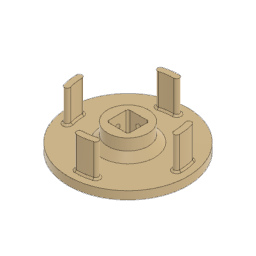
spool adapter v11 (Autodesk Fusion 360 design; units mm, degrees)
Autodesk Fusion 360 part; units mm, degrees
note: some values were not read from the file. Set by a fixed rule: which sketch regions a step uses.
sketch "Sketch1" plane through (0, 0, 0) normal (0, 0, 1) x (1, 0, 0)
  circle A0 centre (0, 0) radius 36.75
  dimension "d1" = 73.5
  constraint coincident A0.centre origin
  measures "d1" diameter of A0
extrude "Extrude1" add sketch "Sketch1" along normal blind 5
sketch "Sketch3" plane through (0, 0, 5) normal (0, 0, 1) x (-1, 0, 0)
  circle A0 centre (0, 0) radius 36.75
  circle A1 centre (0, 0) radius 30 construction
  line L0 (0, 0) -> (-30, 0) construction
  arc A2 (-31.75, 0) -> (-30.3627, -9.2828) centre (0, 0) ccw
  arc A3 (-28.25, 0) -> (-31.75, 0) centre (-30, 0) ccw
  arc A4 (-28.25, 0) -> (-27.0156, -8.2595) centre (0, 0) ccw
  arc A5 (-30.3627, -9.2828) -> (-27.0156, -8.2595) centre (-28.6891, -8.7712) ccw
  arc A6 (-30, 0) -> (-28.6891, -8.7712) centre (0, 0) ccw construction
  dimension "d8" = 60
  dimension "d24" = 3.5
  dimension "d27" = 17
  constraint coincident A0.centre A1.centre
  constraint coincident A1 L0.end
  constraint horizontal L0
  constraint tangent A2 A3
  constraint tangent A3 A4
  constraint tangent A4 A5
  constraint tangent A2 A5
  constraint coincident L0.end A3.centre
  measures "d8" diameter of A1
  measures "d24" distance of A2 A4
  measures "d27" angle of A5.centre L0.end A0.centre
extrude "Extrude3" add sketch "Sketch3" along normal blind 20 contours A2 A3 A4 A5
chamfer "Chamfer2" distance 1 angle 45 4 edges at (27.9397, 4.1756, 5) (28.1775, 10.4447, 5) (31.4013, 4.6929, 5) (30, -1.75, 5)
pattern_circular "C-Pattern1" count 4 over 360 about axis through (0, 0, 1.75) along (0, 0, 1) of "Extrude3", "Chamfer2"
sketch "Sketch4" plane through (0, 0, 5) normal (0, 0, 1) x (-1, 0, 0)
  circle A0 centre (0, 0) radius 12.5
  arc A1 (27.25, 0) -> (26.0593, 7.9671) centre (0, 0) ccw
  arc A2 (31.319, 9.5752) -> (26.0593, 7.9671) centre (28.6891, 8.7712) ccw
  arc A3 (27.25, 0) -> (32.75, 0) centre (30, 0) ccw
  arc A4 (-27.25, 0) -> (-26.0593, -7.9671) centre (0, 0) ccw
  arc A5 (-31.319, -9.5752) -> (-26.0593, -7.9671) centre (-28.6891, -8.7712) ccw
  arc A6 (-27.25, 0) -> (-32.75, 0) centre (-30, 0) ccw
  arc A7 (0, -27.25) -> (7.9671, -26.0593) centre (0, 0) ccw
  arc A8 (9.5752, -31.319) -> (7.9671, -26.0593) centre (8.7712, -28.6891) ccw
  arc A9 (0, -27.25) -> (0, -32.75) centre (0, -30) ccw
  arc A10 (0, 27.25) -> (-7.9671, 26.0593) centre (0, 0) ccw
  arc A11 (-9.5752, 31.319) -> (-7.9671, 26.0593) centre (-8.7712, 28.6891) ccw
  arc A12 (0, 27.25) -> (0, 32.75) centre (0, 30) ccw
  arc A13 (32.75, 0) -> (31.319, 9.5752) centre (0, 0) ccw
  arc A14 (-32.75, 0) -> (-31.319, -9.5752) centre (0, 0) ccw
  circle A15 centre (0, 0) radius 36.75
  arc A16 (0, -32.75) -> (9.5752, -31.319) centre (0, 0) ccw
  arc A17 (0, 32.75) -> (-9.5752, 31.319) centre (0, 0) ccw
  dimension "d14" = 25
  constraint coincident A0.centre A1.centre
  measures "d14" diameter of A0
extrude "Extrude4" add sketch "Sketch4" along normal blind 11 contours A0
sketch "Sketch5" plane through (0, 0, 0) normal (0, 0, -1) x (1, 0, 0)
  circle A0 centre (0, 0) radius 36.75
  line L0 (6.6, -6.6) -> (-6.6, -6.6)
  line L1 (-6.6, -6.6) -> (-6.6, 6.6)
  line L2 (-6.6, 6.6) -> (6.6, 6.6)
  line L3 (6.6, 6.6) -> (6.6, -6.6)
  line L4 (6.6, -6.6) -> (-6.6, 6.6) construction
  line L5 (-6.6, -6.6) -> (6.6, 6.6) construction
  dimension "d17" = 13.2
  dimension "d18" = 13.2
  constraint perpendicular L0 L1
  constraint parallel L0 L2
  constraint parallel L1 L3
  constraint horizontal L0
  constraint coincident L4 A0.centre
  constraint coincident L5 A0.centre
  constraint coincident A0.centre origin
  measures "d17" distance of L0.end L1.end
  measures "d18" distance of L1.end L2.end
extrude "Extrude5" cut sketch "Sketch5" against normal up to surface (16 mm away) contours L0 L1 L2 L3
sketch "Sketch9" plane through (6.5, 0, 0) normal (-1, 0, 0) x (0, -1, 0)
  line L0 (6.5, 19) -> (-6.5, 19)
  line L1 (-6.5, 19) -> (-6.5, 0)
  line L2 (-6.5, 0) -> (6.5, 0)
  line L3 (6.5, 0) -> (6.5, 19)
  line L4 (0, 0) -> (0, 11.85)
  circle A0 centre (0, 9.6) radius 2.25
  dimension "d53" = 9.6
  dimension "d54" = 4.5
  constraint coincident L4.start origin
  constraint perpendicular L2 L4
  constraint coincident L4 A0.centre
  constraint coincident L4.end A0
  measures "d53" distance of L4.start A0.centre
  measures "d54" diameter of A0
revolve "Revolve2" [suppressed]
pattern_circular "C-Pattern3" [suppressed]
sketch "Sketch8" plane through (0, 0, 0) normal (0, 0, -1) x (1, 0, 0)
  line L0 (6.6, 6.6) -> (6.6, -6.6)
  line L1 (6.6, -6.6) -> (-6.6, -6.6)
  line L2 (-6.6, -6.6) -> (-6.6, 6.6)
  line L3 (-6.6, 6.6) -> (6.6, 6.6)
  circle A0 centre (0, 0) radius 36.75
  circle A1 centre (0, 0) radius 7.75
  dimension "d49" = 15.5
  constraint coincident A0.centre A1.centre
  measures "d49" diameter of A1
extrude "Extrude8" cut sketch "Sketch8" against normal blind 10 draft -30 contours L0 A1 | L0 L1 L2 L3 A1 | L3 A1 | L1 A1 | L2 A1
fillet "Fillet2" radius 1.3 4 edges at (-6.6, 6.6, 8) (6.6, -6.6, 8) (-6.6, -6.6, 8) (6.6, 6.6, 8)
chamfer "Chamfer1" distance 4 angle 45 1 edges at (11.6541, -4.5202, 5)
ref_plane "WorkPlane1" through (5.6, 0, 8) normal (-1, 0, 0) x (0, -1, 0)
sketch "Sketch10" plane through (5.6, 0, 9.5) normal (-1, 0, 0) x (0, 1, 0)
  line L0 (5.3, -6.5) -> (5.3, 9.5)
  line L1 (5.3, 9.5) -> (4.0623, 9.5)
  spline S0 degree 2 poles (4.0623, 9.5) (0, 5.8118) (-4.0623, 9.5) knots 0 0 0 0.904876 0.904876 0.904876 weights 1 1.174242 1
  line L2 (-4.0623, 9.5) -> (-5.3, 9.5)
  line L3 (-5.3, 9.5) -> (-5.3, -6.5)
  line L4 (-5.3, -6.5) -> (5.3, -6.5)
  spline S1 degree 2 poles (4.0623, 9.5) (0, 5.8118) (-4.0623, 9.5) knots 0 0 0 0.904876 0.904876 0.904876 weights 1 1.174242 1
  line L5 (-4.0623, 9.5) -> (4.0623, 9.5)
  line L6 (0, 9.5) -> (0, -6.5)
  circle A0 centre (0, 0) radius 2
  dimension "d60" = 4
  dimension "d61" = 9.5
  constraint midpoint L5 L6.start
  constraint midpoint L4 L6.end
  constraint coincident L6 A0.centre
  measures "d60" diameter of A0
  measures "d61" distance of L5 A0.centre
revolve "Revolve3" cut sketch "Sketch10" angle 360 about axis through (5.6, 0, 0) along (0, 0, 1) contours L6 A0 picked at (0.5315, 0.497)
pattern_circular "C-Pattern4" count 4 over 360 about axis through (0, 0, 1.75) along (0, 0, 1) of "Revolve3"
equation "d1 = id + 2 * wall + 2 * 5 mm"
equation "d8 = id + wall"
equation "d12 = tab_length"
equation "d17 = d18"
equation "id = 56.5 mm"
equation "wall = 3.5 mm"
equation "d24 = wall"
equation "d27 = angle"
equation "angle = 17 deg"
equation "n = 4"
equation "tab_length = 20 mm"
